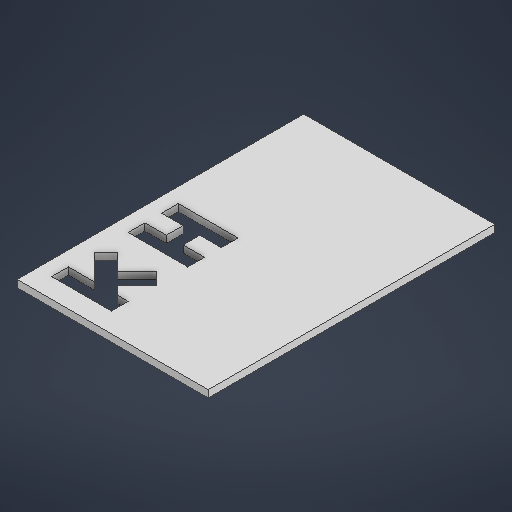
# Autodesk Inventor part: lazer
Saved by Autodesk Inventor 2026 (Build 300175000, 175)
## iProperties
Created: 2025-09-29
Part Number: lazer
Material: Generic
Document SubType Name: Modeling
Designer: 7019505
Density: 1 g/cm^3
Appearance: Default
Author: 7019505
Autodesk Inventor part; units mm, degrees
ref_plane "YZ Plane" through (0, 0, 0) normal (1, 0, 0) x (0, 1, 0)
ref_plane "XZ Plane" through (0, 0, 0) normal (0, 1, 0) x (-1, 0, 0)
ref_plane "XY Plane" through (0, 0, 0) normal (0, 0, 1) x (1, 0, 0)
sketch "Sketch1" plane through (0, 0, 0) normal (0, 1, 0) x (-1, 0, 0)
  line L0 (0, 0) -> (80, 0)
  line L1 (80, 0) -> (80, -120)
  line L2 (80, -120) -> (0, -120)
  line L3 (0, -120) -> (0, 0)
  line L4 (73.8042, -8.2645) -> (48.8042, -8.2645)
  line L5 (48.8042, -8.2645) -> (48.8042, -15.2645)
  line L6 (73.8042, -15.2645) -> (73.8042, -8.2645)
  line L7 (63.0542, -15.2645) -> (66.5542, -15.2645)
  line L8 (63.0542, -15.2645) -> (73.8042, -26.0145)
  line L9 (63.0542, -15.2645) -> (78.257, -15.2645) construction
  line L10 (73.8042, -26.0145) -> (68.8545, -30.9642)
  line L11 (56.867, -18.9768) -> (54.3922, -16.5019)
  line L12 (56.867, -18.9768) -> (48.8042, -27.0396)
  line L13 (56.867, -18.9768) -> (68.2696, -18.9768) construction
  line L14 (48.8042, -27.0396) -> (53.754, -31.9894)
  line L15 (53.754, -31.9894) -> (61.8168, -23.9265)
  line L16 (68.8545, -30.9642) -> (61.8168, -23.9265)
  line L17 (56.867, -18.9768) -> (53.1547, -15.2645)
  line L18 (48.8042, -15.2645) -> (53.1547, -15.2645)
  line L19 (63.0542, -15.2645) -> (73.8042, -15.2645)
  line L20 (48.8042, -40.2645) -> (73.8042, -40.2645)
  line L21 (73.8042, -40.2645) -> (73.8042, -47.2645)
  line L22 (73.8042, -47.2645) -> (64.8042, -47.2645)
  line L23 (64.8042, -47.2645) -> (64.8042, -54.2645)
  line L24 (64.8042, -54.2645) -> (73.8042, -54.2645)
  line L25 (73.8042, -54.2645) -> (73.8042, -61.2645)
  line L26 (73.8042, -61.2645) -> (48.8042, -61.2645)
  line L27 (48.8042, -61.2645) -> (48.8042, -54.2645)
  line L28 (48.8042, -54.2645) -> (57.8042, -54.2645)
  line L29 (57.8042, -54.2645) -> (57.8042, -47.2645)
  line L30 (57.8042, -47.2645) -> (48.8042, -47.2645)
  line L31 (48.8042, -47.2645) -> (48.8042, -40.2645)
  dimension "d0" = 80
  dimension "d1" = 120
  dimension "d2" = 80
  dimension "d41" = 25
  dimension "d42" = 7
  dimension "d43" = 25
  dimension "d44" = 3.5
  dimension "d45" = 45
  dimension "d46" = 7
  dimension "d47" = 3.5
  dimension "d48" = 135
  dimension "d49" = 7
  dimension "d50" = 7
  dimension "d51" = 9
  dimension "d52" = 7
  dimension "d53" = 9
  dimension "d54" = 7
  dimension "d55" = 7
  dimension "d56" = 9
  dimension "d57" = 7
  dimension "d58" = 9
  constraints: 64 end point, 14 perpendicular, 8 point on line, 6 horizontal, 2 equal length, 1 parallel
  measures "d0" distance of L0.start L0.end
  measures "d1" distance of L0.end L1.end
  measures "d2" distance of L1.end L2.end
  measures "d41" distance of L4.start L4.end
  measures "d42" distance of L4.end L5.end
  measures "d43" distance of L5.end L6.start
  measures "d44" distance of L7.start L7.end
  measures "d45" angle of L8 L9
  measures "d46" distance of L8.end L10.end
  measures "d47" distance of L11.start L11.end
  measures "d48" angle of L12 L13
  measures "d49" distance of L12.end L14.end
  measures "d50" distance of L20.end L21.end
  measures "d51" distance of L21.end L22.end
  measures "d52" distance of L22.end L23.end
  measures "d53" distance of L23.end L24.end
  measures "d54" distance of L24.end L25.end
  measures "d55" distance of L26.end L27.end
  measures "d56" distance of L27.end L28.end
  measures "d57" distance of L28.end L29.end
  measures "d58" distance of L29.end L30.end
extrude "Extrusion1" add sketch "Sketch1" along normal blind 3 contours L0 L1 L2 L3 | L6 L19 L7 L8 L10 L16 L15 L14 L12 L11 L17 L18 L5 L4 | L20 L21 L22 L23 L24 L25 L26 L27 L28 L29 L30 L31
extrude "Extrusion2" cut sketch "Sketch1" along normal blind 50.5 contours L6 L19 L7 L8 L10 L16 L15 L14 L12 L11 L17 L18 L5 L4 | L20 L21 L22 L23 L24 L25 L26 L27 L28 L29 L30 L31
body "Solid1"
